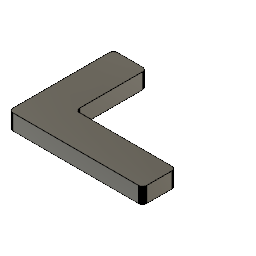
Ell (Autodesk Fusion 360 design; units mm, degrees)
Autodesk Fusion 360 part; units mm, degrees
sketch "Sketch1" plane through (0, 0, 0) normal (0, 0, 1) x (1, 0, 0)
  line L0 (22.6961, -14.7008) -> (22.7107, -14.7004)
  line L1 (22.7107, -14.7004) -> (22.7254, -14.6998)
  line L2 (22.7254, -14.6998) -> (22.74, -14.6989)
  line L3 (22.74, -14.6989) -> (22.7546, -14.6977)
  line L4 (22.7546, -14.6977) -> (22.7692, -14.6963)
  line L5 (22.7692, -14.6963) -> (22.7838, -14.6946)
  line L6 (22.7838, -14.6946) -> (22.7983, -14.6927)
  line L7 (22.7983, -14.6927) -> (22.8128, -14.6906)
  line L8 (22.8128, -14.6906) -> (22.8273, -14.6882)
  line L9 (22.8273, -14.6882) -> (22.8417, -14.6855)
  line L10 (22.8417, -14.6855) -> (22.8561, -14.6825)
  line L11 (22.8561, -14.6825) -> (22.8704, -14.6794)
  line L12 (22.8704, -14.6794) -> (22.8846, -14.676)
  line L13 (22.8846, -14.676) -> (22.8988, -14.6723)
  line L14 (22.8988, -14.6723) -> (22.9129, -14.6684)
  line L15 (22.9129, -14.6684) -> (22.927, -14.6642)
  line L16 (22.927, -14.6642) -> (22.941, -14.6598)
  line L17 (22.941, -14.6598) -> (22.9549, -14.6551)
  line L18 (22.9549, -14.6551) -> (22.9687, -14.6502)
  line L19 (22.9687, -14.6502) -> (22.9824, -14.6451)
  line L20 (22.9824, -14.6451) -> (22.9961, -14.6397)
  line L21 (22.9961, -14.6397) -> (23.0096, -14.6341)
  line L22 (23.0096, -14.6341) -> (23.0231, -14.6283)
  line L23 (23.0231, -14.6283) -> (23.0364, -14.6222)
  line L24 (23.0364, -14.6222) -> (23.0497, -14.6159)
  line L25 (23.0497, -14.6159) -> (23.0628, -14.6093)
  line L26 (23.0628, -14.6093) -> (23.0758, -14.6026)
  line L27 (23.0758, -14.6026) -> (23.0887, -14.5956)
  line L28 (23.0887, -14.5956) -> (23.1014, -14.5884)
  line L29 (23.1014, -14.5884) -> (23.1141, -14.5809)
  line L30 (23.1141, -14.5809) -> (23.1266, -14.5733)
  line L31 (23.1266, -14.5733) -> (23.1389, -14.5654)
  line L32 (23.1389, -14.5654) -> (23.1511, -14.5573)
  line L33 (23.1511, -14.5573) -> (23.1632, -14.549)
  line L34 (23.1632, -14.549) -> (23.1752, -14.5405)
  line L35 (23.1752, -14.5405) -> (23.187, -14.5318)
  line L36 (23.187, -14.5318) -> (23.1986, -14.5228)
  line L37 (23.1986, -14.5228) -> (23.2101, -14.5137)
  line L38 (23.2101, -14.5137) -> (23.2214, -14.5044)
  line L39 (23.2214, -14.5044) -> (23.2325, -14.4949)
  line L40 (23.2325, -14.4949) -> (23.2435, -14.4851)
  line L41 (23.2435, -14.4851) -> (23.2543, -14.4752)
  line L42 (23.2543, -14.4752) -> (23.2649, -14.4651)
  line L43 (23.2649, -14.4651) -> (23.2754, -14.4549)
  line L44 (23.2754, -14.4549) -> (23.2857, -14.4444)
  line L45 (23.2857, -14.4444) -> (23.2958, -14.4338)
  line L46 (23.2958, -14.4338) -> (23.3057, -14.423)
  line L47 (23.3057, -14.423) -> (23.3154, -14.412)
  line L48 (23.3154, -14.412) -> (23.3249, -14.4008)
  line L49 (23.3249, -14.4008) -> (23.3342, -14.3895)
  line L50 (23.3342, -14.3895) -> (23.3434, -14.378)
  line L51 (23.3434, -14.378) -> (23.3523, -14.3664)
  line L52 (23.3523, -14.3664) -> (23.361, -14.3546)
  line L53 (23.361, -14.3546) -> (23.3695, -14.3427)
  line L54 (23.3695, -14.3427) -> (23.3778, -14.3306)
  line L55 (23.3778, -14.3306) -> (23.3859, -14.3184)
  line L56 (23.3859, -14.3184) -> (23.3938, -14.306)
  line L57 (23.3938, -14.306) -> (23.4015, -14.2935)
  line L58 (23.4015, -14.2935) -> (23.4089, -14.2809)
  line L59 (23.4089, -14.2809) -> (23.4161, -14.2681)
  line L60 (23.4161, -14.2681) -> (23.4231, -14.2552)
  line L61 (23.4231, -14.2552) -> (23.4299, -14.2422)
  line L62 (23.4299, -14.2422) -> (23.4364, -14.2291)
  line L63 (23.4364, -14.2291) -> (23.4427, -14.2159)
  line L64 (23.4427, -14.2159) -> (23.4488, -14.2025)
  line L65 (23.4488, -14.2025) -> (23.4547, -14.1891)
  line L66 (23.4547, -14.1891) -> (23.4603, -14.1756)
  line L67 (23.4603, -14.1756) -> (23.4657, -14.1619)
  line L68 (23.4657, -14.1619) -> (23.4708, -14.1482)
  line L69 (23.4708, -14.1482) -> (23.4757, -14.1344)
  line L70 (23.4757, -14.1344) -> (23.4803, -14.1204)
  line L71 (23.4803, -14.1204) -> (23.4848, -14.1065)
  line L72 (23.4848, -14.1065) -> (23.4889, -14.0924)
  line L73 (23.4889, -14.0924) -> (23.4928, -14.0783)
  line L74 (23.4928, -14.0783) -> (23.4965, -14.0641)
  line L75 (23.4965, -14.0641) -> (23.4999, -14.0498)
  line L76 (23.4999, -14.0498) -> (23.5031, -14.0355)
  line L77 (23.5031, -14.0355) -> (23.506, -14.0211)
  line L78 (23.506, -14.0211) -> (23.5087, -14.0067)
  line L79 (23.5087, -14.0067) -> (23.5111, -13.9923)
  line L80 (23.5111, -13.9923) -> (23.5133, -13.9778)
  line L81 (23.5133, -13.9778) -> (23.5152, -13.9632)
  line L82 (23.5152, -13.9632) -> (23.5169, -13.9487)
  line L83 (23.5169, -13.9487) -> (23.5183, -13.9341)
  line L84 (23.5183, -13.9341) -> (23.5194, -13.9195)
  line L85 (23.5194, -13.9195) -> (23.5203, -13.9048)
  line L86 (23.5203, -13.9048) -> (23.521, -13.8902)
  line L87 (23.521, -13.8902) -> (23.5213, -13.8755)
  line L88 (23.5213, -13.8755) -> (23.5215, -13.8609)
  line L89 (23.5215, -13.8609) -> (23.5215, -8.8205)
  line L90 (23.5215, -8.8205) -> (23.5213, -8.8059)
  line L91 (23.5213, -8.8059) -> (23.521, -8.7912)
  line L92 (23.521, -8.7912) -> (23.5203, -8.7766)
  line L93 (23.5203, -8.7766) -> (23.5194, -8.7619)
  line L94 (23.5194, -8.7619) -> (23.5183, -8.7473)
  line L95 (23.5183, -8.7473) -> (23.5169, -8.7327)
  line L96 (23.5169, -8.7327) -> (23.5152, -8.7182)
  line L97 (23.5152, -8.7182) -> (23.5133, -8.7036)
  line L98 (23.5133, -8.7036) -> (23.5111, -8.6891)
  line L99 (23.5111, -8.6891) -> (23.5087, -8.6747)
  line L100 (23.5087, -8.6747) -> (23.506, -8.6603)
  line L101 (23.506, -8.6603) -> (23.5031, -8.6459)
  line L102 (23.5031, -8.6459) -> (23.4999, -8.6316)
  line L103 (23.4999, -8.6316) -> (23.4965, -8.6173)
  line L104 (23.4965, -8.6173) -> (23.4928, -8.6031)
  line L105 (23.4928, -8.6031) -> (23.4889, -8.589)
  line L106 (23.4889, -8.589) -> (23.4848, -8.5749)
  line L107 (23.4848, -8.5749) -> (23.4803, -8.561)
  line L108 (23.4803, -8.561) -> (23.4757, -8.547)
  line L109 (23.4757, -8.547) -> (23.4708, -8.5332)
  line L110 (23.4708, -8.5332) -> (23.4657, -8.5195)
  line L111 (23.4657, -8.5195) -> (23.4603, -8.5059)
  line L112 (23.4603, -8.5059) -> (23.4547, -8.4923)
  line L113 (23.4547, -8.4923) -> (23.4488, -8.4789)
  line L114 (23.4488, -8.4789) -> (23.4427, -8.4655)
  line L115 (23.4427, -8.4655) -> (23.4364, -8.4523)
  line L116 (23.4364, -8.4523) -> (23.4299, -8.4392)
  line L117 (23.4299, -8.4392) -> (23.4231, -8.4262)
  line L118 (23.4231, -8.4262) -> (23.4161, -8.4133)
  line L119 (23.4161, -8.4133) -> (23.4089, -8.4005)
  line L120 (23.4089, -8.4005) -> (23.4015, -8.3879)
  line L121 (23.4015, -8.3879) -> (23.3938, -8.3754)
  line L122 (23.3938, -8.3754) -> (23.3859, -8.363)
  line L123 (23.3859, -8.363) -> (23.3778, -8.3508)
  line L124 (23.3778, -8.3508) -> (23.3695, -8.3387)
  line L125 (23.3695, -8.3387) -> (23.361, -8.3268)
  line L126 (23.361, -8.3268) -> (23.3523, -8.315)
  line L127 (23.3523, -8.315) -> (23.3434, -8.3034)
  line L128 (23.3434, -8.3034) -> (23.3342, -8.2919)
  line L129 (23.3342, -8.2919) -> (23.3249, -8.2806)
  line L130 (23.3249, -8.2806) -> (23.3154, -8.2694)
  line L131 (23.3154, -8.2694) -> (23.3057, -8.2584)
  line L132 (23.3057, -8.2584) -> (23.2958, -8.2476)
  line L133 (23.2958, -8.2476) -> (23.2857, -8.237)
  line L134 (23.2857, -8.237) -> (23.2754, -8.2265)
  line L135 (23.2754, -8.2265) -> (23.2649, -8.2163)
  line L136 (23.2649, -8.2163) -> (23.2543, -8.2062)
  line L137 (23.2543, -8.2062) -> (23.2435, -8.1963)
  line L138 (23.2435, -8.1963) -> (23.2325, -8.1866)
  line L139 (23.2325, -8.1866) -> (23.2214, -8.177)
  line L140 (23.2214, -8.177) -> (23.2101, -8.1677)
  line L141 (23.2101, -8.1677) -> (23.1986, -8.1586)
  line L142 (23.1986, -8.1586) -> (23.187, -8.1496)
  line L143 (23.187, -8.1496) -> (23.1752, -8.1409)
  line L144 (23.1752, -8.1409) -> (23.1632, -8.1324)
  line L145 (23.1632, -8.1324) -> (23.1511, -8.1241)
  line L146 (23.1511, -8.1241) -> (23.1389, -8.116)
  line L147 (23.1389, -8.116) -> (23.1266, -8.1082)
  line L148 (23.1266, -8.1082) -> (23.1141, -8.1005)
  line L149 (23.1141, -8.1005) -> (23.1014, -8.093)
  line L150 (23.1014, -8.093) -> (23.0887, -8.0858)
  line L151 (23.0887, -8.0858) -> (23.0758, -8.0788)
  line L152 (23.0758, -8.0788) -> (23.0628, -8.0721)
  line L153 (23.0628, -8.0721) -> (23.0497, -8.0655)
  line L154 (23.0497, -8.0655) -> (23.0364, -8.0592)
  line L155 (23.0364, -8.0592) -> (23.0231, -8.0531)
  line L156 (23.0231, -8.0531) -> (23.0096, -8.0473)
  line L157 (23.0096, -8.0473) -> (22.9961, -8.0417)
  line L158 (22.9961, -8.0417) -> (22.9824, -8.0363)
  line L159 (22.9824, -8.0363) -> (22.9687, -8.0312)
  line L160 (22.9687, -8.0312) -> (22.9549, -8.0263)
  line L161 (22.9549, -8.0263) -> (22.941, -8.0216)
  line L162 (22.941, -8.0216) -> (22.927, -8.0172)
  line L163 (22.927, -8.0172) -> (22.9129, -8.013)
  line L164 (22.9129, -8.013) -> (22.8988, -8.0091)
  line L165 (22.8988, -8.0091) -> (22.8846, -8.0054)
  line L166 (22.8846, -8.0054) -> (22.8704, -8.002)
  line L167 (22.8704, -8.002) -> (22.8561, -7.9989)
  line L168 (22.8561, -7.9989) -> (22.8417, -7.9959)
  line L169 (22.8417, -7.9959) -> (22.8273, -7.9932)
  line L170 (22.8273, -7.9932) -> (22.8128, -7.9908)
  line L171 (22.8128, -7.9908) -> (22.7983, -7.9887)
  line L172 (22.7983, -7.9887) -> (22.7838, -7.9868)
  line L173 (22.7838, -7.9868) -> (22.7692, -7.9851)
  line L174 (22.7692, -7.9851) -> (22.7546, -7.9837)
  line L175 (22.7546, -7.9837) -> (22.74, -7.9825)
  line L176 (22.74, -7.9825) -> (22.7254, -7.9817)
  line L177 (22.7254, -7.9817) -> (22.7107, -7.981)
  line L178 (22.7107, -7.981) -> (22.6961, -7.9806)
  line L179 (22.6961, -7.9806) -> (22.6814, -7.9805)
  line L180 (22.6814, -7.9805) -> (4.204, -7.9805)
  line L181 (4.204, -7.9805) -> (4.1857, -7.9803)
  line L182 (4.1857, -7.9803) -> (4.171, -7.9799)
  line L183 (4.171, -7.9799) -> (4.1561, -7.9793)
  line L184 (4.1561, -7.9793) -> (4.1417, -7.9784)
  line L185 (4.1417, -7.9784) -> (4.127, -7.9773)
  line L186 (4.127, -7.9773) -> (4.1126, -7.9759)
  line L187 (4.1126, -7.9759) -> (4.0979, -7.9742)
  line L188 (4.0979, -7.9742) -> (4.0833, -7.9723)
  line L189 (4.0833, -7.9723) -> (4.0689, -7.9701)
  line L190 (4.0689, -7.9701) -> (4.0543, -7.9677)
  line L191 (4.0543, -7.9677) -> (4.0399, -7.965)
  line L192 (4.0399, -7.965) -> (4.0257, -7.9621)
  line L193 (4.0257, -7.9621) -> (4.0113, -7.959)
  line L194 (4.0113, -7.959) -> (3.9968, -7.9555)
  line L195 (3.9968, -7.9555) -> (3.9829, -7.9519)
  line L196 (3.9829, -7.9519) -> (3.9688, -7.9479)
  line L197 (3.9688, -7.9479) -> (3.9547, -7.9438)
  line L198 (3.9547, -7.9438) -> (3.9408, -7.9394)
  line L199 (3.9408, -7.9394) -> (3.9268, -7.9347)
  line L200 (3.9268, -7.9347) -> (3.913, -7.9298)
  line L201 (3.913, -7.9298) -> (3.8991, -7.9246)
  line L202 (3.8991, -7.9246) -> (3.8857, -7.9193)
  line L203 (3.8857, -7.9193) -> (3.872, -7.9137)
  line L204 (3.872, -7.9137) -> (3.8586, -7.9079)
  line L205 (3.8586, -7.9079) -> (3.8452, -7.9017)
  line L206 (3.8452, -7.9017) -> (3.832, -7.8954)
  line L207 (3.832, -7.8954) -> (3.8188, -7.8889)
  line L208 (3.8188, -7.8889) -> (3.8061, -7.8822)
  line L209 (3.8061, -7.8822) -> (3.7929, -7.8751)
  line L210 (3.7929, -7.8751) -> (3.7803, -7.868)
  line L211 (3.7803, -7.868) -> (3.7676, -7.8605)
  line L212 (3.7676, -7.8605) -> (3.755, -7.8528)
  line L213 (3.755, -7.8528) -> (3.7428, -7.8449)
  line L214 (3.7428, -7.8449) -> (3.7305, -7.8369)
  line L215 (3.7305, -7.8369) -> (3.7185, -7.8286)
  line L216 (3.7185, -7.8286) -> (3.7064, -7.82)
  line L217 (3.7064, -7.82) -> (3.6947, -7.8113)
  line L218 (3.6947, -7.8113) -> (3.683, -7.8024)
  line L219 (3.683, -7.8024) -> (3.6716, -7.7932)
  line L220 (3.6716, -7.7932) -> (3.6604, -7.784)
  line L221 (3.6604, -7.784) -> (3.6491, -7.7744)
  line L222 (3.6491, -7.7744) -> (3.6382, -7.7647)
  line L223 (3.6382, -7.7647) -> (3.6273, -7.7547)
  line L224 (3.6273, -7.7547) -> (3.6167, -7.7447)
  line L225 (3.6167, -7.7447) -> (3.6063, -7.7344)
  line L226 (3.6063, -7.7344) -> (3.596, -7.724)
  line L227 (3.596, -7.724) -> (3.586, -7.7134)
  line L228 (3.586, -7.7134) -> (3.576, -7.7025)
  line L229 (3.576, -7.7025) -> (3.5663, -7.6916)
  line L230 (3.5663, -7.6916) -> (3.5567, -7.6803)
  line L231 (3.5567, -7.6803) -> (3.5475, -7.6691)
  line L232 (3.5475, -7.6691) -> (3.5384, -7.6577)
  line L233 (3.5384, -7.6577) -> (3.5294, -7.646)
  line L234 (3.5294, -7.646) -> (3.5207, -7.6343)
  line L235 (3.5207, -7.6343) -> (3.5121, -7.6222)
  line L236 (3.5121, -7.6222) -> (3.5039, -7.6102)
  line L237 (3.5039, -7.6102) -> (3.4958, -7.5979)
  line L238 (3.4958, -7.5979) -> (3.4879, -7.5857)
  line L239 (3.4879, -7.5857) -> (3.4802, -7.5731)
  line L240 (3.4802, -7.5731) -> (3.4727, -7.5604)
  line L241 (3.4727, -7.5604) -> (3.4656, -7.5478)
  line L242 (3.4656, -7.5478) -> (3.4585, -7.5346)
  line L243 (3.4585, -7.5346) -> (3.4518, -7.5219)
  line L244 (3.4518, -7.5219) -> (3.4453, -7.5087)
  line L245 (3.4453, -7.5087) -> (3.439, -7.4955)
  line L246 (3.439, -7.4955) -> (3.4328, -7.4821)
  line L247 (3.4328, -7.4821) -> (3.427, -7.4687)
  line L248 (3.427, -7.4687) -> (3.4214, -7.455)
  line L249 (3.4214, -7.455) -> (3.4161, -7.4416)
  line L250 (3.4161, -7.4416) -> (3.4109, -7.4277)
  line L251 (3.4109, -7.4277) -> (3.406, -7.4139)
  line L252 (3.406, -7.4139) -> (3.4013, -7.3999)
  line L253 (3.4013, -7.3999) -> (3.3969, -7.386)
  line L254 (3.3969, -7.386) -> (3.3928, -7.372)
  line L255 (3.3928, -7.372) -> (3.3888, -7.3578)
  line L256 (3.3888, -7.3578) -> (3.3852, -7.3439)
  line L257 (3.3852, -7.3439) -> (3.3817, -7.3294)
  line L258 (3.3817, -7.3294) -> (3.3786, -7.315)
  line L259 (3.3786, -7.315) -> (3.3757, -7.3008)
  line L260 (3.3757, -7.3008) -> (3.373, -7.2864)
  line L261 (3.373, -7.2864) -> (3.3706, -7.2718)
  line L262 (3.3706, -7.2718) -> (3.3684, -7.2574)
  line L263 (3.3684, -7.2574) -> (3.3665, -7.2428)
  line L264 (3.3665, -7.2428) -> (3.3648, -7.2282)
  line L265 (3.3648, -7.2282) -> (3.3634, -7.2137)
  line L266 (3.3634, -7.2137) -> (3.3623, -7.199)
  line L267 (3.3623, -7.199) -> (3.3614, -7.1846)
  line L268 (3.3614, -7.1846) -> (3.3608, -7.1697)
  line L269 (3.3608, -7.1697) -> (3.3604, -7.155)
  line L270 (3.3604, -7.155) -> (3.3602, -7.1367)
  line L271 (3.3602, -7.1367) -> (3.3602, 5.4603)
  line L272 (3.3602, 5.4603) -> (3.3601, 5.475)
  line L273 (3.3601, 5.475) -> (3.3597, 5.4897)
  line L274 (3.3597, 5.4897) -> (3.359, 5.5043)
  line L275 (3.359, 5.5043) -> (3.3582, 5.5189)
  line L276 (3.3582, 5.5189) -> (3.357, 5.5335)
  line L277 (3.357, 5.5335) -> (3.3556, 5.5482)
  line L278 (3.3556, 5.5482) -> (3.3539, 5.5627)
  line L279 (3.3539, 5.5627) -> (3.352, 5.5773)
  line L280 (3.352, 5.5773) -> (3.3499, 5.5918)
  line L281 (3.3499, 5.5918) -> (3.3475, 5.6062)
  line L282 (3.3475, 5.6062) -> (3.3448, 5.6206)
  line L283 (3.3448, 5.6206) -> (3.3418, 5.635)
  line L284 (3.3418, 5.635) -> (3.3387, 5.6493)
  line L285 (3.3387, 5.6493) -> (3.3353, 5.6636)
  line L286 (3.3353, 5.6636) -> (3.3316, 5.6777)
  line L287 (3.3316, 5.6777) -> (3.3277, 5.6919)
  line L288 (3.3277, 5.6919) -> (3.3235, 5.706)
  line L289 (3.3235, 5.706) -> (3.3191, 5.7199)
  line L290 (3.3191, 5.7199) -> (3.3144, 5.7338)
  line L291 (3.3144, 5.7338) -> (3.3095, 5.7476)
  line L292 (3.3095, 5.7476) -> (3.3044, 5.7614)
  line L293 (3.3044, 5.7614) -> (3.299, 5.775)
  line L294 (3.299, 5.775) -> (3.2934, 5.7886)
  line L295 (3.2934, 5.7886) -> (3.2876, 5.802)
  line L296 (3.2876, 5.802) -> (3.2815, 5.8154)
  line L297 (3.2815, 5.8154) -> (3.2752, 5.8286)
  line L298 (3.2752, 5.8286) -> (3.2686, 5.8417)
  line L299 (3.2686, 5.8417) -> (3.2619, 5.8547)
  line L300 (3.2619, 5.8547) -> (3.2549, 5.8676)
  line L301 (3.2549, 5.8676) -> (3.2477, 5.8804)
  line L302 (3.2477, 5.8804) -> (3.2402, 5.893)
  line L303 (3.2402, 5.893) -> (3.2325, 5.9055)
  line L304 (3.2325, 5.9055) -> (3.2247, 5.9179)
  line L305 (3.2247, 5.9179) -> (3.2166, 5.9301)
  line L306 (3.2166, 5.9301) -> (3.2083, 5.9422)
  line L307 (3.2083, 5.9422) -> (3.1998, 5.9541)
  line L308 (3.1998, 5.9541) -> (3.1911, 5.9659)
  line L309 (3.1911, 5.9659) -> (3.1821, 5.9775)
  line L310 (3.1821, 5.9775) -> (3.173, 5.989)
  line L311 (3.173, 5.989) -> (3.1637, 6.0003)
  line L312 (3.1637, 6.0003) -> (3.1542, 6.0115)
  line L313 (3.1542, 6.0115) -> (3.1444, 6.0224)
  line L314 (3.1444, 6.0224) -> (3.1345, 6.0332)
  line L315 (3.1345, 6.0332) -> (3.1244, 6.0439)
  line L316 (3.1244, 6.0439) -> (3.1142, 6.0544)
  line L317 (3.1142, 6.0544) -> (3.1037, 6.0646)
  line L318 (3.1037, 6.0646) -> (3.0931, 6.0747)
  line L319 (3.0931, 6.0747) -> (3.0823, 6.0846)
  line L320 (3.0823, 6.0846) -> (3.0713, 6.0943)
  line L321 (3.0713, 6.0943) -> (3.0601, 6.1039)
  line L322 (3.0601, 6.1039) -> (3.0488, 6.1132)
  line L323 (3.0488, 6.1132) -> (3.0373, 6.1223)
  line L324 (3.0373, 6.1223) -> (3.0257, 6.1312)
  line L325 (3.0257, 6.1312) -> (3.0139, 6.1399)
  line L326 (3.0139, 6.1399) -> (3.002, 6.1485)
  line L327 (3.002, 6.1485) -> (2.9899, 6.1568)
  line L328 (2.9899, 6.1568) -> (2.9777, 6.1649)
  line L329 (2.9777, 6.1649) -> (2.9653, 6.1727)
  line L330 (2.9653, 6.1727) -> (2.9528, 6.1804)
  line L331 (2.9528, 6.1804) -> (2.9402, 6.1878)
  line L332 (2.9402, 6.1878) -> (2.9274, 6.1951)
  line L333 (2.9274, 6.1951) -> (2.9145, 6.2021)
  line L334 (2.9145, 6.2021) -> (2.9015, 6.2088)
  line L335 (2.9015, 6.2088) -> (2.8884, 6.2154)
  line L336 (2.8884, 6.2154) -> (2.8752, 6.2217)
  line L337 (2.8752, 6.2217) -> (2.8618, 6.2278)
  line L338 (2.8618, 6.2278) -> (2.8484, 6.2336)
  line L339 (2.8484, 6.2336) -> (2.8349, 6.2392)
  line L340 (2.8349, 6.2392) -> (2.8212, 6.2446)
  line L341 (2.8212, 6.2446) -> (2.8075, 6.2497)
  line L342 (2.8075, 6.2497) -> (2.7937, 6.2546)
  line L343 (2.7937, 6.2546) -> (2.7797, 6.2593)
  line L344 (2.7797, 6.2593) -> (2.7658, 6.2637)
  line L345 (2.7658, 6.2637) -> (2.7517, 6.2678)
  line L346 (2.7517, 6.2678) -> (2.7376, 6.2718)
  line L347 (2.7376, 6.2718) -> (2.7234, 6.2754)
  line L348 (2.7234, 6.2754) -> (2.7091, 6.2789)
  line L349 (2.7091, 6.2789) -> (2.6948, 6.282)
  line L350 (2.6948, 6.282) -> (2.6804, 6.285)
  line L351 (2.6804, 6.285) -> (2.666, 6.2876)
  line L352 (2.666, 6.2876) -> (2.6516, 6.29)
  line L353 (2.6516, 6.29) -> (2.6371, 6.2922)
  line L354 (2.6371, 6.2922) -> (2.6225, 6.2941)
  line L355 (2.6225, 6.2941) -> (2.608, 6.2958)
  line L356 (2.608, 6.2958) -> (2.5934, 6.2972)
  line L357 (2.5934, 6.2972) -> (2.5788, 6.2984)
  line L358 (2.5788, 6.2984) -> (2.5641, 6.2993)
  line L359 (2.5641, 6.2993) -> (2.5495, 6.2999)
  line L360 (2.5495, 6.2999) -> (2.5348, 6.3003)
  line L361 (2.5348, 6.3003) -> (2.5202, 6.3004)
  line L362 (2.5202, 6.3004) -> (-2.5202, 6.3004)
  line L363 (-2.5202, 6.3004) -> (-2.5348, 6.3003)
  line L364 (-2.5348, 6.3003) -> (-2.5495, 6.2999)
  line L365 (-2.5495, 6.2999) -> (-2.5641, 6.2993)
  line L366 (-2.5641, 6.2993) -> (-2.5788, 6.2984)
  line L367 (-2.5788, 6.2984) -> (-2.5934, 6.2972)
  line L368 (-2.5934, 6.2972) -> (-2.608, 6.2958)
  line L369 (-2.608, 6.2958) -> (-2.6225, 6.2941)
  line L370 (-2.6225, 6.2941) -> (-2.6371, 6.2922)
  line L371 (-2.6371, 6.2922) -> (-2.6516, 6.29)
  line L372 (-2.6516, 6.29) -> (-2.666, 6.2876)
  line L373 (-2.666, 6.2876) -> (-2.6804, 6.285)
  line L374 (-2.6804, 6.285) -> (-2.6948, 6.282)
  line L375 (-2.6948, 6.282) -> (-2.7091, 6.2789)
  line L376 (-2.7091, 6.2789) -> (-2.7234, 6.2754)
  line L377 (-2.7234, 6.2754) -> (-2.7376, 6.2718)
  line L378 (-2.7376, 6.2718) -> (-2.7517, 6.2678)
  line L379 (-2.7517, 6.2678) -> (-2.7658, 6.2637)
  line L380 (-2.7658, 6.2637) -> (-2.7797, 6.2593)
  line L381 (-2.7797, 6.2593) -> (-2.7937, 6.2546)
  line L382 (-2.7937, 6.2546) -> (-2.8075, 6.2497)
  line L383 (-2.8075, 6.2497) -> (-2.8212, 6.2446)
  line L384 (-2.8212, 6.2446) -> (-2.8349, 6.2392)
  line L385 (-2.8349, 6.2392) -> (-2.8484, 6.2336)
  line L386 (-2.8484, 6.2336) -> (-2.8618, 6.2278)
  line L387 (-2.8618, 6.2278) -> (-2.8752, 6.2217)
  line L388 (-2.8752, 6.2217) -> (-2.8884, 6.2154)
  line L389 (-2.8884, 6.2154) -> (-2.9015, 6.2088)
  line L390 (-2.9015, 6.2088) -> (-2.9145, 6.2021)
  line L391 (-2.9145, 6.2021) -> (-2.9274, 6.1951)
  line L392 (-2.9274, 6.1951) -> (-2.9402, 6.1878)
  line L393 (-2.9402, 6.1878) -> (-2.9528, 6.1804)
  line L394 (-2.9528, 6.1804) -> (-2.9653, 6.1727)
  line L395 (-2.9653, 6.1727) -> (-2.9777, 6.1649)
  line L396 (-2.9777, 6.1649) -> (-2.9899, 6.1568)
  line L397 (-2.9899, 6.1568) -> (-3.002, 6.1485)
  line L398 (-3.002, 6.1485) -> (-3.0139, 6.1399)
  line L399 (-3.0139, 6.1399) -> (-3.0257, 6.1312)
  line L400 (-3.0257, 6.1312) -> (-3.0373, 6.1223)
  line L401 (-3.0373, 6.1223) -> (-3.0488, 6.1132)
  line L402 (-3.0488, 6.1132) -> (-3.0601, 6.1039)
  line L403 (-3.0601, 6.1039) -> (-3.0713, 6.0943)
  line L404 (-3.0713, 6.0943) -> (-3.0823, 6.0846)
  line L405 (-3.0823, 6.0846) -> (-3.0931, 6.0747)
  line L406 (-3.0931, 6.0747) -> (-3.1037, 6.0646)
  line L407 (-3.1037, 6.0646) -> (-3.1142, 6.0544)
  line L408 (-3.1142, 6.0544) -> (-3.1244, 6.0439)
  line L409 (-3.1244, 6.0439) -> (-3.1345, 6.0332)
  line L410 (-3.1345, 6.0332) -> (-3.1444, 6.0224)
  line L411 (-3.1444, 6.0224) -> (-3.1542, 6.0115)
  line L412 (-3.1542, 6.0115) -> (-3.1637, 6.0003)
  line L413 (-3.1637, 6.0003) -> (-3.173, 5.989)
  line L414 (-3.173, 5.989) -> (-3.1821, 5.9775)
  line L415 (-3.1821, 5.9775) -> (-3.1911, 5.9659)
  line L416 (-3.1911, 5.9659) -> (-3.1998, 5.9541)
  line L417 (-3.1998, 5.9541) -> (-3.2083, 5.9422)
  line L418 (-3.2083, 5.9422) -> (-3.2166, 5.9301)
  line L419 (-3.2166, 5.9301) -> (-3.2247, 5.9179)
  line L420 (-3.2247, 5.9179) -> (-3.2325, 5.9055)
  line L421 (-3.2325, 5.9055) -> (-3.2402, 5.893)
  line L422 (-3.2402, 5.893) -> (-3.2477, 5.8804)
  line L423 (-3.2477, 5.8804) -> (-3.2549, 5.8676)
  line L424 (-3.2549, 5.8676) -> (-3.2619, 5.8547)
  line L425 (-3.2619, 5.8547) -> (-3.2686, 5.8417)
  line L426 (-3.2686, 5.8417) -> (-3.2752, 5.8286)
  line L427 (-3.2752, 5.8286) -> (-3.2815, 5.8154)
  line L428 (-3.2815, 5.8154) -> (-3.2876, 5.802)
  line L429 (-3.2876, 5.802) -> (-3.2934, 5.7886)
  line L430 (-3.2934, 5.7886) -> (-3.299, 5.775)
  line L431 (-3.299, 5.775) -> (-3.3044, 5.7614)
  line L432 (-3.3044, 5.7614) -> (-3.3095, 5.7476)
  line L433 (-3.3095, 5.7476) -> (-3.3144, 5.7338)
  line L434 (-3.3144, 5.7338) -> (-3.3191, 5.7199)
  line L435 (-3.3191, 5.7199) -> (-3.3235, 5.706)
  line L436 (-3.3235, 5.706) -> (-3.3277, 5.6919)
  line L437 (-3.3277, 5.6919) -> (-3.3316, 5.6777)
  line L438 (-3.3316, 5.6777) -> (-3.3353, 5.6636)
  line L439 (-3.3353, 5.6636) -> (-3.3387, 5.6493)
  line L440 (-3.3387, 5.6493) -> (-3.3418, 5.635)
  line L441 (-3.3418, 5.635) -> (-3.3448, 5.6206)
  line L442 (-3.3448, 5.6206) -> (-3.3475, 5.6062)
  line L443 (-3.3475, 5.6062) -> (-3.3499, 5.5918)
  line L444 (-3.3499, 5.5918) -> (-3.352, 5.5773)
  line L445 (-3.352, 5.5773) -> (-3.3539, 5.5627)
  line L446 (-3.3539, 5.5627) -> (-3.3556, 5.5482)
  line L447 (-3.3556, 5.5482) -> (-3.357, 5.5335)
  line L448 (-3.357, 5.5335) -> (-3.3582, 5.5189)
  line L449 (-3.3582, 5.5189) -> (-3.3591, 5.5043)
  line L450 (-3.3591, 5.5043) -> (-3.3597, 5.4897)
  line L451 (-3.3597, 5.4897) -> (-3.3601, 5.475)
  line L452 (-3.3601, 5.475) -> (-3.3602, 5.4603)
  line L453 (-3.3602, 5.4603) -> (-3.3602, -13.8609)
  line L454 (-3.3602, -13.8609) -> (-3.3601, -13.8755)
  line L455 (-3.3601, -13.8755) -> (-3.3597, -13.8902)
  line L456 (-3.3597, -13.8902) -> (-3.3591, -13.9048)
  line L457 (-3.3591, -13.9048) -> (-3.3582, -13.9195)
  line L458 (-3.3582, -13.9195) -> (-3.357, -13.9341)
  line L459 (-3.357, -13.9341) -> (-3.3556, -13.9487)
  line L460 (-3.3556, -13.9487) -> (-3.3539, -13.9632)
  line L461 (-3.3539, -13.9632) -> (-3.352, -13.9778)
  line L462 (-3.352, -13.9778) -> (-3.3499, -13.9923)
  line L463 (-3.3499, -13.9923) -> (-3.3475, -14.0067)
  line L464 (-3.3475, -14.0067) -> (-3.3448, -14.0211)
  line L465 (-3.3448, -14.0211) -> (-3.3418, -14.0355)
  line L466 (-3.3418, -14.0355) -> (-3.3387, -14.0498)
  line L467 (-3.3387, -14.0498) -> (-3.3353, -14.0641)
  line L468 (-3.3353, -14.0641) -> (-3.3316, -14.0783)
  line L469 (-3.3316, -14.0783) -> (-3.3277, -14.0924)
  line L470 (-3.3277, -14.0924) -> (-3.3235, -14.1065)
  line L471 (-3.3235, -14.1065) -> (-3.3191, -14.1204)
  line L472 (-3.3191, -14.1204) -> (-3.3144, -14.1344)
  line L473 (-3.3144, -14.1344) -> (-3.3095, -14.1482)
  line L474 (-3.3095, -14.1482) -> (-3.3044, -14.1619)
  line L475 (-3.3044, -14.1619) -> (-3.299, -14.1756)
  line L476 (-3.299, -14.1756) -> (-3.2934, -14.1891)
  line L477 (-3.2934, -14.1891) -> (-3.2876, -14.2025)
  line L478 (-3.2876, -14.2025) -> (-3.2815, -14.2159)
  line L479 (-3.2815, -14.2159) -> (-3.2752, -14.2291)
  line L480 (-3.2752, -14.2291) -> (-3.2686, -14.2422)
  line L481 (-3.2686, -14.2422) -> (-3.2619, -14.2552)
  line L482 (-3.2619, -14.2552) -> (-3.2549, -14.2681)
  line L483 (-3.2549, -14.2681) -> (-3.2477, -14.2809)
  line L484 (-3.2477, -14.2809) -> (-3.2402, -14.2935)
  line L485 (-3.2402, -14.2935) -> (-3.2325, -14.306)
  line L486 (-3.2325, -14.306) -> (-3.2247, -14.3184)
  line L487 (-3.2247, -14.3184) -> (-3.2166, -14.3306)
  line L488 (-3.2166, -14.3306) -> (-3.2083, -14.3427)
  line L489 (-3.2083, -14.3427) -> (-3.1998, -14.3546)
  line L490 (-3.1998, -14.3546) -> (-3.1911, -14.3664)
  line L491 (-3.1911, -14.3664) -> (-3.1821, -14.378)
  line L492 (-3.1821, -14.378) -> (-3.173, -14.3895)
  line L493 (-3.173, -14.3895) -> (-3.1637, -14.4008)
  line L494 (-3.1637, -14.4008) -> (-3.1542, -14.412)
  line L495 (-3.1542, -14.412) -> (-3.1444, -14.423)
  line L496 (-3.1444, -14.423) -> (-3.1345, -14.4338)
  line L497 (-3.1345, -14.4338) -> (-3.1244, -14.4444)
  line L498 (-3.1244, -14.4444) -> (-3.1142, -14.4549)
  line L499 (-3.1142, -14.4549) -> (-3.1037, -14.4651)
  line L500 (-3.1037, -14.4651) -> (-3.0931, -14.4752)
  line L501 (-3.0931, -14.4752) -> (-3.0823, -14.4851)
  line L502 (-3.0823, -14.4851) -> (-3.0713, -14.4949)
  line L503 (-3.0713, -14.4949) -> (-3.0601, -14.5044)
  line L504 (-3.0601, -14.5044) -> (-3.0488, -14.5137)
  line L505 (-3.0488, -14.5137) -> (-3.0373, -14.5228)
  line L506 (-3.0373, -14.5228) -> (-3.0257, -14.5318)
  line L507 (-3.0257, -14.5318) -> (-3.0139, -14.5405)
  line L508 (-3.0139, -14.5405) -> (-3.002, -14.549)
  line L509 (-3.002, -14.549) -> (-2.9899, -14.5573)
  line L510 (-2.9899, -14.5573) -> (-2.9777, -14.5654)
  line L511 (-2.9777, -14.5654) -> (-2.9653, -14.5733)
  line L512 (-2.9653, -14.5733) -> (-2.9528, -14.5809)
  line L513 (-2.9528, -14.5809) -> (-2.9402, -14.5884)
  line L514 (-2.9402, -14.5884) -> (-2.9274, -14.5956)
  line L515 (-2.9274, -14.5956) -> (-2.9145, -14.6026)
  line L516 (-2.9145, -14.6026) -> (-2.9015, -14.6093)
  line L517 (-2.9015, -14.6093) -> (-2.8884, -14.6159)
  line L518 (-2.8884, -14.6159) -> (-2.8752, -14.6222)
  line L519 (-2.8752, -14.6222) -> (-2.8618, -14.6283)
  line L520 (-2.8618, -14.6283) -> (-2.8484, -14.6341)
  line L521 (-2.8484, -14.6341) -> (-2.8349, -14.6397)
  line L522 (-2.8349, -14.6397) -> (-2.8212, -14.6451)
  line L523 (-2.8212, -14.6451) -> (-2.8075, -14.6502)
  line L524 (-2.8075, -14.6502) -> (-2.7937, -14.6551)
  line L525 (-2.7937, -14.6551) -> (-2.7797, -14.6598)
  line L526 (-2.7797, -14.6598) -> (-2.7658, -14.6642)
  line L527 (-2.7658, -14.6642) -> (-2.7517, -14.6684)
  line L528 (-2.7517, -14.6684) -> (-2.7376, -14.6723)
  line L529 (-2.7376, -14.6723) -> (-2.7234, -14.676)
  line L530 (-2.7234, -14.676) -> (-2.7091, -14.6794)
  line L531 (-2.7091, -14.6794) -> (-2.6948, -14.6825)
  line L532 (-2.6948, -14.6825) -> (-2.6804, -14.6855)
  line L533 (-2.6804, -14.6855) -> (-2.666, -14.6882)
  line L534 (-2.666, -14.6882) -> (-2.6516, -14.6906)
  line L535 (-2.6516, -14.6906) -> (-2.6371, -14.6927)
  line L536 (-2.6371, -14.6927) -> (-2.6225, -14.6946)
  line L537 (-2.6225, -14.6946) -> (-2.608, -14.6963)
  line L538 (-2.608, -14.6963) -> (-2.5934, -14.6977)
  line L539 (-2.5934, -14.6977) -> (-2.5788, -14.6989)
  line L540 (-2.5788, -14.6989) -> (-2.5641, -14.6998)
  line L541 (-2.5641, -14.6998) -> (-2.5495, -14.7004)
  line L542 (-2.5495, -14.7004) -> (-2.5348, -14.7008)
  line L543 (-2.5348, -14.7008) -> (-2.5202, -14.7009)
  line L544 (-2.5202, -14.7009) -> (22.6814, -14.7009)
  line L545 (22.6814, -14.7009) -> (22.6961, -14.7008)
extrude "Extrude1" add sketch "Sketch1" along normal blind 3.175
